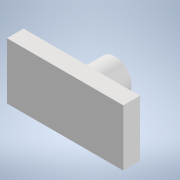
# Autodesk Inventor part: z axis base
Saved by Autodesk Inventor 2021 (Build 250183000, 183)
## iProperties
Created: 2021-05-05
Part Number: z axis base
Material: Generic
Document SubType Name: Modeling
Designer: techv
Density: 1 g/cm^3
Appearance: Default
Author: techv
Autodesk Inventor part; units mm, degrees
ref_plane "YZ Plane" through (0, 0, 0) normal (1, 0, 0) x (0, 1, 0)
ref_plane "XZ Plane" through (0, 0, 0) normal (0, 1, 0) x (-1, 0, 0)
ref_plane "XY Plane" through (0, 0, 0) normal (0, 0, 1) x (1, 0, 0)
sketch "Sketch1" plane through (0, 0, 0) normal (0, 0, 1) x (1, 0, 0)
  circle A0 centre (0, 0) radius 5
  arc A1 (-1.5, -2) -> (-1.5, 2) centre (0, 0) ccw projected
  line L0 (-1.5, 2) -> (-1.5, -2) projected
  dimension "d0" = 10
  constraints: 1 centre point, 1 coincident
  measures "d0" diameter of A0
extrude "Extrusion1" add sketch "Sketch1" against normal blind 10
sketch "Sketch2" plane through (0, 0, 0) normal (0, 0, 1) x (1, 0, 0)
  line L0 (-17.5, 8.5) -> (17.5, 8.5)
  line L1 (17.5, 8.5) -> (17.5, -8.5)
  line L2 (17.5, -8.5) -> (-17.5, -8.5)
  line L3 (-17.5, -8.5) -> (-17.5, 8.5)
  line L4 (-17.5, 8.5) -> (17.5, -8.5) construction
  line L5 (17.5, 8.5) -> (-17.5, -8.5) construction
  point P0 (0, 0)
  dimension "d3" = 35
  dimension "d4" = 17
  constraints: 12 end point, 2 midpoint, 2 parallel, 1 horizontal, 1 perpendicular
  measures "d3" distance of L1.end L2.end
  measures "d4" distance of L0.end L1.end
extrude "Extrusion2" add sketch "Sketch2" along normal blind 5
sketch "Sketch3" plane through (-17.5, -8.5, 0) normal (-1, 0, 0) x (0, 0, 1)
  line L0 (0, 0) -> (5, 0) projected
  line L1 (5, 0) -> (5, 17) projected
  line L2 (0, 0) -> (5, 0)
  line L3 (5, 0) -> (5, 17)
  line L4 (5, 17) -> (0, 17)
  line L5 (0, 17) -> (0, 0)
  point P0 (0, 8.5)
  constraints: 8 end point, 2 parallel, 1 horizontal, 1 perpendicular
extrude "Extrusion3" add sketch "Sketch3" along normal blind 45
sketch "Sketch4" plane through (17.5, -8.5, 0) normal (1, 0, 0) x (0, 0, -1)
  line L0 (0, 0) -> (0, 17) projected
  line L1 (-5, 0) -> (-5, 17) projected
  line L2 (0, 0) -> (-5, 0)
  line L3 (-5, 0) -> (-5, 17)
  line L4 (-5, 17) -> (0, 17)
  line L5 (0, 17) -> (0, 0)
  point P0 (0, 8.5)
  constraints: 8 end point, 2 parallel, 1 horizontal, 1 perpendicular
extrude "Extrusion4" add sketch "Sketch4" along normal blind 45
sketch "Sketch5" plane through (0, 0, 5) normal (0, 0, 1) x (1, 0, 0)
  line L0 (62.5, -8.5) -> (-62.5, -8.5) projected
  line L1 (62.5, -8.5) -> (57.5, -8.5)
  line L2 (57.5, -8.5) -> (57.5, 8.5)
  line L3 (57.5, 8.5) -> (62.5, 8.5)
  line L4 (62.5, 8.5) -> (62.5, -8.5)
  point P0 (0, 0)
  dimension "d11" = 5
  dimension "d12" = 17
  constraints: 8 end point, 2 parallel, 1 horizontal, 1 perpendicular
  measures "d11" distance of L2.end L3.end
  measures "d12" distance of L1.end L2.end
extrude "Extrusion5" add sketch "Sketch5" along normal blind 17
sketch "Sketch6" plane through (0, 0, 5) normal (0, 0, 1) x (1, 0, 0)
  line L0 (-62.5, -8.5) -> (62.5, -8.5) projected
  line L1 (-62.5, 8.5) -> (-57.5, 8.5)
  line L2 (-57.5, 8.5) -> (-57.5, -8.5)
  line L3 (-57.5, -8.5) -> (-62.5, -8.5)
  line L4 (-62.5, -8.5) -> (-62.5, 8.5)
  point P0 (0, 0)
  dimension "d15" = 5
  constraints: 8 end point, 2 parallel, 1 horizontal, 1 perpendicular, 1 point on line
  measures "d15" distance of L2.end L3.end
extrude "Extrusion6" add sketch "Sketch6" along normal blind 17
sketch "Sketch7" plane through (-62.5, -8.5, 0) normal (-1, 0, 0) x (0, 0, 1)
  line L0 (0, 0) -> (22, 0) projected
  line L1 (22, 0) -> (5, 0)
  line L2 (5, 0) -> (5, 17)
  line L3 (5, 17) -> (22, 17)
  line L4 (22, 17) -> (22, 0)
  line L5 (5, 17) -> (22, 0)
  line L6 (5, 0) -> (22, 17)
  circle A0 centre (13.5, 8.5) radius 1.5
  point P0 (0, 8.5)
  dimension "d18" = 17
  dimension "d19" = 17
  dimension "d20" = 3
  constraints: 12 end point, 2 parallel, 1 centre point, 1 horizontal, 1 midpoint, 1 perpendicular
  measures "d18" distance of L2.end L3.end
  measures "d19" distance of L1.end L2.end
  measures "d20" diameter of A0
extrude "Extrusion7" cut sketch "Sketch7" against normal through all contours A0 L5 L6 | L6 L5 A0 | L5 L6 A0 | A0 L6 L5
body "Solid1"
